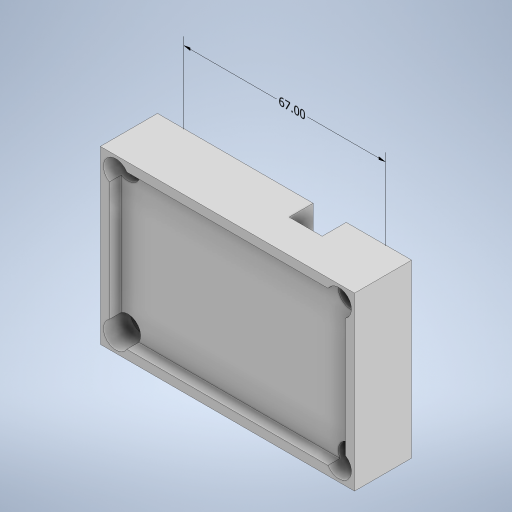
# Autodesk Inventor part: bms_case
Saved by Autodesk Inventor 2023 (Build 270158000, 158)
## iProperties
Created: 2024-04-17
Part Number: bms_case
Material: Genérico
Document SubType Name: Modeling
Designer: inigo
Density: 1 g/cm^3
Appearance: Valor por defecto
Author: inigo
Autodesk Inventor part; units mm, degrees
ref_plane "YZ Plane" through (0, 0, 0) normal (1, 0, 0) x (0, 1, 0)
ref_plane "XZ Plane" through (0, 0, 0) normal (0, 1, 0) x (-1, 0, 0)
ref_plane "XY Plane" through (0, 0, 0) normal (0, 0, 1) x (1, 0, 0)
sketch "Boceto1" plane through (0, 0, 0) normal (0, 0, 1) x (1, 0, 0)
  line L0 (-39.25, 25.5) -> (39.25, 25.5)
  line L1 (39.25, 25.5) -> (39.25, -25.5)
  line L2 (39.25, -25.5) -> (-39.25, -25.5)
  line L3 (-39.25, -25.5) -> (-39.25, 25.5)
  line L4 (-39.25, 25.5) -> (39.25, -25.5) construction
  line L5 (39.25, 25.5) -> (-39.25, -25.5) construction
  line L6 (42.25, 28.5) -> (-42.25, 28.5)
  line L7 (-42.25, 28.5) -> (-42.25, -28.5)
  line L8 (-42.25, -28.5) -> (42.25, -28.5)
  line L9 (42.25, -28.5) -> (42.25, 28.5)
  point P0 (0, 0)
  dimension "d0" = 51
  dimension "d1" = 78.5
  dimension "d2" = 3
  constraints: 20 end point, 4 parallel, 2 midpoint, 2 perpendicular, 1 horizontal, 3 other
  measures "d0" distance of L0.end L1.end
  measures "d1" distance between parallel lines of L3 L1
  measures "d2" distance between parallel lines of L0 L6
extrude "Extrusión1" add sketch "Boceto1" along normal blind 4
sketch "Boceto2" plane through (0, 0, 0) normal (0, 0, -1) x (-1, 0, 0)
  line L0 (-42.25, 28.5) -> (42.25, 28.5) projected
  line L1 (42.25, -28.5) -> (-42.25, -28.5) projected
  line L2 (-42.25, 28.5) -> (42.25, 28.5)
  line L3 (42.25, 28.5) -> (42.25, -28.5)
  line L4 (42.25, -28.5) -> (-42.25, -28.5)
  line L5 (-42.25, -28.5) -> (-42.25, 28.5)
  point P0 (0, 0)
  point P1 (-42.25, -28.5)
  constraints: 8 end point, 2 parallel, 1 horizontal, 1 perpendicular
extrude "Extrusión2" add sketch "Boceto2" along normal blind 15
sketch "Boceto3" plane through (0, 0, -15) normal (0, 0, -1) x (-1, 0, 0)
  line L0 (-33.5, 17.5) -> (33.5, 17.5)
  line L1 (33.5, 17.5) -> (33.5, -17.5)
  line L2 (33.5, -17.5) -> (-33.5, -17.5)
  line L3 (-33.5, -17.5) -> (-33.5, 17.5)
  line L4 (-33.5, 17.5) -> (33.5, -17.5) construction
  line L5 (33.5, 17.5) -> (-33.5, -17.5) construction
  line L6 (31.0225, -10) -> (35.9775, -10)
  line L7 (35.9775, -10) -> (35.9775, 10)
  line L8 (35.9775, 10) -> (31.0225, 10)
  line L9 (31.0225, 10) -> (31.0225, -10)
  line L10 (31.0225, -10) -> (35.9775, 10) construction
  line L11 (35.9775, -10) -> (31.0225, 10) construction
  line L12 (33.5, 10) -> (42.25, 10)
  line L13 (42.25, 28.5) -> (42.25, -28.5) projected
  line L14 (33.5, -10) -> (42.25, -10)
  line L15 (42.25, -10) -> (42.25, 10)
  line L16 (-20.5, 20.388) -> (-9.5, 20.388)
  line L17 (-9.5, 20.388) -> (-9.5, 14.612)
  line L18 (-9.5, 14.612) -> (-20.5, 14.612)
  line L19 (-20.5, 14.612) -> (-20.5, 20.388)
  line L20 (-20.5, 20.388) -> (-9.5, 14.612) construction
  line L21 (-9.5, 20.388) -> (-20.5, 14.612) construction
  line L22 (-42.25, 28.5) -> (42.25, 28.5) projected
  line L23 (-20.5, 17.5) -> (-9.5, 17.5)
  line L24 (-9.5, 17.5) -> (-9.5, 28.5)
  line L25 (-9.5, 28.5) -> (-20.5, 28.5)
  line L26 (-20.5, 28.5) -> (-20.5, 17.5)
  line L27 (-33.5, 0) -> (-37.4386, 0)
  line L28 (-20.5, -20.388) -> (-9.5, -20.388)
  line L29 (-9.5, -20.388) -> (-9.5, -14.612)
  line L30 (-9.5, -14.612) -> (-20.5, -14.612)
  line L31 (-20.5, -14.612) -> (-20.5, -20.388)
  line L32 (-20.5, -20.388) -> (-9.5, -14.612) construction
  line L33 (-9.5, -20.388) -> (-20.5, -14.612) construction
  line L34 (-20.5, -17.5) -> (-9.5, -17.5)
  line L35 (-9.5, -17.5) -> (-9.5, -28.5)
  line L36 (-9.5, -28.5) -> (-20.5, -28.5)
  line L37 (-20.5, -28.5) -> (-20.5, -17.5)
  point P0 (0, 0)
  point P1 (33.5, 0)
  point P2 (33.5, 10)
  point P3 (-15, 17.5)
  point P4 (-15, -17.5)
  point P5 (-20.5, -17.5)
  point P6 (-9.5, -17.5)
  point P7 (-20.5, 28.5)
  point P8 (-20.5, 17.5)
  point P9 (-9.5, 17.5)
  dimension "d7" = 67
  dimension "d8" = 35
  dimension "d9" = 20
  dimension "d33" = 11
  dimension "d34" = 13
  dimension "d38" = 0
  constraints: 72 end point, 11 midpoint, 9 symmetric about line, 8 parallel, 7 horizontal, 5 perpendicular, 3 point on line
  measures "d7" distance of L1.end L2.end
  measures "d8" distance of L0.end L1.end
  measures "d9" distance of L7.end L6.end
  measures "d33" distance of L17.end L18.end
  measures "d34" distance between parallel lines of L3 L19
  measures "d38" distance between parallel lines of L17 L24
extrude "Extrusión3" cut sketch "Boceto3" against normal blind 8 contours L0 L19 L18 L17 L1 L8 L9 L6 L2 L29 L30 L31 L3 | L19 L16 L17 L0 | L0 L17 L18 L19 | L26 L22 L24 L16 | L31 L30 L29 L2 | L2 L29 L28 L31 | L8 L7 L6 L1 | L1 L6 L9 L8 | L28 L35 L36 L37 | L12 L13 L14 L7
sketch "Boceto4" plane through (0, 0, 0) normal (0, 0, 1) x (1, 0, 0)
  line L0 (-42.05, -28.35) -> (-42.05, 28.35)
  line L1 (-42.05, 28.35) -> (42.05, 28.35)
  line L2 (42.05, 28.35) -> (42.05, -28.35)
  line L3 (42.05, -28.35) -> (-42.05, -28.35)
  line L4 (-42.05, -28.35) -> (42.05, 28.35) construction
  line L5 (-42.05, 28.35) -> (42.05, -28.35) construction
  line L6 (10.704, 28.35) -> (-32.296, 28.35)
  line L7 (42.05, 8.05) -> (42.05, 12.05)
  circle A0 centre (-37.05, -23.35) radius 2.25
  line L8 (-42.05, 12.05) -> (-42.05, -12.05)
  line L9 (-42.05, 0) -> (-48.6371, 0)
  line L10 (0, -28.35) -> (0, -35.954)
  circle A1 centre (-37.05, 23.35) radius 2.25
  circle A2 centre (37.05, -23.35) radius 2.25
  circle A3 centre (37.05, 23.35) radius 2.25
  point P0 (0, 0)
  point P1 (0, 0)
  dimension "d12" = 0
  dimension "d13" = 0
  dimension "d14" = 4.5
  dimension "d15" = 5
  dimension "d16" = 5
  dimension "d24" = 4.5
  dimension "d25" = 4.5
  dimension "d26" = 4.5
  constraints: 22 end point, 4 centre point, 4 midpoint, 3 symmetric about line, 2 parallel, 1 perpendicular, 3 other
  measures "d12" distance between parallel lines of L6 L1
  measures "d13" distance between parallel lines of L7 L2
  measures "d14" diameter of A0
  measures "d15" distance from line of L0 A0.centre
  measures "d16" distance from line of L3 A0.centre
  measures "d24" diameter of A1
  measures "d25" diameter of A3
  measures "d26" diameter of A2
extrude "Extrusión4" cut sketch "Boceto4" against normal blind 15 contours A0 | A1 | A2 | A3
sketch "Boceto5" plane through (0, 0, 0) normal (0, 0, 1) x (1, 0, 0)
  circle A0 centre (-37.05, 23.35) radius 2.25 projected
  line L0 (-39.25, 25.5) -> (39.25, 25.5) projected
  arc A1 (39.25, 23.8217) -> (37.7133, 25.5) centre (37.05, 23.35) ccw projected
  circle A2 centre (37.05, 23.35) radius 2.5
  circle A3 centre (37.05, -23.35) radius 2.25 projected
  circle A4 centre (37.05, -23.35) radius 2.15
  line L1 (39.25, -25.5) -> (-39.25, -25.5) projected
  arc A5 (-36.3867, -25.5) -> (-39.25, -22.8783) centre (-37.05, -23.35) ccw projected
  circle A6 centre (-37.05, -23.35) radius 2.5
  circle A7 centre (-37.05, 23.35) radius 2.5
  circle A8 centre (37.05, -23.35) radius 2.5
  point P0 (0, 0)
  dimension "d28" = 5
  dimension "d29" = 4.5
  dimension "d30" = 5
  dimension "d31" = 5
  dimension "d32" = 5
  constraints: 5 centre point, 5 coincident, 1 tangent
  measures "d28" diameter of A2
  measures "d29" diameter of A3
  measures "d30" diameter of A6
  measures "d31" diameter of A7
  measures "d32" diameter of A8
extrude "Extrusión5" cut sketch "Boceto5" against normal blind 5 contours A2 L0 | L0 A2 | A4 | A6 L1 | L1 A6
sketch "Boceto6" plane through (-37.05, 23.35, -5) normal (0, 0, 1) x (1, 0, 0)
  circle A0 centre (0, 0) radius 4.2
  line L0 (37.05, 4.6715) -> (37.05, 10.9086)
  line L1 (-5.2, -13.35) -> (-5.2, -33.35) projected
  line L2 (-5.2, -23.35) -> (-13.3544, -23.35)
  circle A1 centre (74.1, 0) radius 4.2
  circle A2 centre (0, -46.7) radius 4.2
  circle A3 centre (74.1, -46.7) radius 4.2
  point P0 (37.05, -23.35)
  dimension "d21" = 8.4
  constraints: 4 centre point, 4 end point, 3 symmetric about line, 1 horizontal, 1 midpoint, 1 vertical, 3 other
  measures "d21" diameter of A0
extrude "Extrusión6" cut sketch "Boceto6" along normal blind 9
